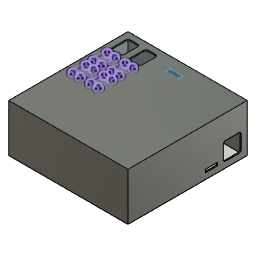
Outer+Hull (Autodesk Fusion 360 design; units mm, degrees)
Autodesk Fusion 360 part; units mm, degrees
sketch "Sketch1" plane through (0, 0, 0) normal (0, 1, 0) x (1, 0, 0) in component "Outer Hull"
  line L0 (0, 0) -> (100, 0)
  line L1 (100, 0) -> (100, -100)
  line L2 (100, -100) -> (0, -100)
  line L3 (0, -100) -> (0, 0)
  dimension "d1" = 100
  dimension "d2" = 100
  constraint horizontal L0
  constraint vertical L1
  constraint horizontal L2
  constraint vertical L3
  constraint coincident L0.start L3.end
  measures "d1" distance of L0.start L0.end
  measures "d2" distance of L0.start L2.end
extrude "Extrude1" add sketch "Sketch1" along normal blind 40 in component "Outer Hull"
shell "Shell1" thickness 1 removed faces 1 at (33.3333, 0, 33.3333) in component "Outer Hull"
sketch "Button hole" plane through (0, 40, 0) normal (0, 1, 0) x (-1, 0, 0)
  line L0 (0, 100) -> (-100, 100)
  line L1 (-100, 100) -> (-100, 0)
  line L2 (-100, 0) -> (0, 0)
  line L3 (0, 0) -> (0, 100)
  line L4 (-7, 5) -> (-13, 5)
  line L5 (-15, 7) -> (-15, 18)
  line L6 (-13, 20) -> (-7, 20)
  line L7 (-5, 18) -> (-5, 7)
  arc A0 (-7, 5) -> (-5, 7) centre (-7, 7) ccw
  arc A1 (-15, 7) -> (-13, 5) centre (-13, 7) ccw
  arc A2 (-13, 20) -> (-15, 18) centre (-13, 18) ccw
  arc A3 (-5, 18) -> (-7, 20) centre (-7, 18) ccw
  dimension "d6" = 2
  constraint horizontal L4
  constraint vertical L5
  constraint horizontal L6
  constraint vertical L7
  constraint tangent L4 A0
  constraint tangent L7 A0
  constraint tangent L4 A1
  constraint tangent L5 A1
  constraint equal A0 A1
  constraint tangent L5 A2
  constraint tangent L6 A2
  constraint equal A0 A2
  constraint tangent L6 A3
  constraint tangent L7 A3
  constraint equal A0 A3
  measures "d6" radius of A0
extrude "Extrude2" cut sketch "Button hole" against normal blind 1 contours L4 L5 L6 L7 A0 A1 A2 A3 in component "Outer Hull"
pattern_linear "R-Pattern1" count 3 spacing 17.5 along (0, 0, 1) count 2 spacing 15 along (1, 0, 0) of "Extrude2" in component "Outer Hull"
sketch "Top toggle" plane through (0, 40, 0) normal (0, 1, 0) x (-1, 0, 0)
  line L0 (-20, 18) -> (-20, 7)
  arc A0 (-22, 5) -> (-20, 7) centre (-22, 7) ccw
  line L1 (-22, 5) -> (-28, 5)
  arc A1 (-30, 7) -> (-28, 5) centre (-28, 7) ccw
  line L2 (-30, 7) -> (-30, 18)
  arc A2 (-28, 20) -> (-30, 18) centre (-28, 18) ccw
  line L3 (-28, 20) -> (-22, 20)
  arc A3 (-20, 18) -> (-22, 20) centre (-22, 18) ccw
  line L4 (-5, 18) -> (-5, 7)
  arc A4 (-7, 5) -> (-5, 7) centre (-7, 7) ccw
  line L5 (-7, 5) -> (-13, 5)
  arc A5 (-15, 7) -> (-13, 5) centre (-13, 7) ccw
  line L6 (-15, 7) -> (-15, 18)
  arc A6 (-13, 20) -> (-15, 18) centre (-13, 18) ccw
  line L7 (-13, 20) -> (-7, 20)
  arc A7 (-5, 18) -> (-7, 20) centre (-7, 18) ccw
  line L8 (0, 100) -> (-100, 100)
  line L9 (-100, 100) -> (-100, 0)
  line L10 (-100, 0) -> (0, 0)
  line L11 (0, 0) -> (0, 100)
  line L12 (-45, 10) -> (-55, 10)
  line L13 (-55, 10) -> (-55, 12.5)
  line L14 (-55, 12.5) -> (-45, 12.5)
  line L15 (-45, 12.5) -> (-45, 10)
  line L16 (-20, 53) -> (-20, 42)
  arc A8 (-22, 40) -> (-20, 42) centre (-22, 42) ccw
  line L17 (-22, 40) -> (-28, 40)
  arc A9 (-30, 42) -> (-28, 40) centre (-28, 42) ccw
  line L18 (-30, 42) -> (-30, 53)
  arc A10 (-28, 55) -> (-30, 53) centre (-28, 53) ccw
  line L19 (-28, 55) -> (-22, 55)
  arc A11 (-20, 53) -> (-22, 55) centre (-22, 53) ccw
  line L20 (-20, 35.5) -> (-20, 24.5)
  arc A12 (-22, 22.5) -> (-20, 24.5) centre (-22, 24.5) ccw
  line L21 (-22, 22.5) -> (-28, 22.5)
  arc A13 (-30, 24.5) -> (-28, 22.5) centre (-28, 24.5) ccw
  line L22 (-30, 24.5) -> (-30, 35.5)
  arc A14 (-28, 37.5) -> (-30, 35.5) centre (-28, 35.5) ccw
  line L23 (-28, 37.5) -> (-22, 37.5)
  arc A15 (-20, 35.5) -> (-22, 37.5) centre (-22, 35.5) ccw
  line L24 (-5, 53) -> (-5, 42)
  arc A16 (-7, 40) -> (-5, 42) centre (-7, 42) ccw
  line L25 (-7, 40) -> (-13, 40)
  arc A17 (-15, 42) -> (-13, 40) centre (-13, 42) ccw
  line L26 (-15, 42) -> (-15, 53)
  arc A18 (-13, 55) -> (-15, 53) centre (-13, 53) ccw
  line L27 (-13, 55) -> (-7, 55)
  arc A19 (-5, 53) -> (-7, 55) centre (-7, 53) ccw
  line L28 (-5, 35.5) -> (-5, 24.5)
  arc A20 (-7, 22.5) -> (-5, 24.5) centre (-7, 24.5) ccw
  line L29 (-7, 22.5) -> (-13, 22.5)
  arc A21 (-15, 24.5) -> (-13, 22.5) centre (-13, 24.5) ccw
  line L30 (-15, 24.5) -> (-15, 35.5)
  arc A22 (-13, 37.5) -> (-15, 35.5) centre (-13, 35.5) ccw
  line L31 (-13, 37.5) -> (-7, 37.5)
  arc A23 (-5, 35.5) -> (-7, 37.5) centre (-7, 35.5) ccw
  dimension "d17" = 10
  dimension "d18" = 2.5
  constraint horizontal L12
  constraint vertical L13
  constraint horizontal L14
  constraint vertical L15
  measures "d17" distance of L12.start L12.end
  measures "d18" distance of L12.start L14.end
extrude "Extrude3" cut sketch "Top toggle" against normal blind 1 contours L12 L13 L14 L15 in component "Outer Hull"
sketch "Wire inlet" plane through (100, 0, 0) normal (1, 0, 0) x (0, 0, -1)
  line L0 (-100, 0) -> (0, 0)
  line L1 (0, 0) -> (0, 40)
  line L2 (0, 40) -> (-100, 40)
  line L3 (-100, 40) -> (-100, 0)
  line L4 (-7, 5) -> (-18, 5)
  line L5 (-20, 7) -> (-20, 18)
  line L6 (-18, 20) -> (-7, 20)
  line L7 (-5, 18) -> (-5, 7)
  arc A0 (-18, 20) -> (-20, 18) centre (-18, 18) ccw
  arc A1 (-5, 18) -> (-7, 20) centre (-7, 18) ccw
  arc A2 (-7, 5) -> (-5, 7) centre (-7, 7) ccw
  arc A3 (-20, 7) -> (-18, 5) centre (-18, 7) ccw
  dimension "d21" = 2
  constraint horizontal L4
  constraint vertical L5
  constraint horizontal L6
  constraint vertical L7
  constraint tangent L5 A0
  constraint tangent L6 A0
  constraint tangent L6 A1
  constraint tangent L7 A1
  constraint equal A0 A1
  constraint tangent L4 A2
  constraint tangent L7 A2
  constraint equal A0 A2
  constraint tangent L4 A3
  constraint tangent L5 A3
  constraint equal A0 A3
  measures "d21" radius of A0
extrude "Extrude4" cut sketch "Wire inlet" against normal blind 1 contours L4 L5 L6 L7 A0 A1 A2 A3 in component "Outer Hull"
sketch "Sketch4" plane through (100, 0, 0) normal (1, 0, 0) x (0, 0, -1)
  line L0 (-20, 7) -> (-20, 18)
  arc A0 (-18, 20) -> (-20, 18) centre (-18, 18) ccw
  line L1 (-18, 20) -> (-7, 20)
  arc A1 (-5, 18) -> (-7, 20) centre (-7, 18) ccw
  line L2 (-5, 18) -> (-5, 7)
  arc A2 (-7, 5) -> (-5, 7) centre (-7, 7) ccw
  line L3 (-7, 5) -> (-18, 5)
  arc A3 (-20, 7) -> (-18, 5) centre (-18, 7) ccw
  line L4 (-100, 0) -> (0, 0)
  line L5 (0, 0) -> (0, 40)
  line L6 (0, 40) -> (-100, 40)
  line L7 (-100, 40) -> (-100, 0)
  line L8 (-25, 5) -> (-35, 5)
  line L9 (-35, 5) -> (-35, 7.5)
  line L10 (-35, 7.5) -> (-25, 7.5)
  line L11 (-25, 7.5) -> (-25, 5)
  dimension "d24" = 10
  dimension "d25" = 2.5
  constraint horizontal L8
  constraint vertical L9
  constraint horizontal L10
  constraint vertical L11
  measures "d24" distance of L8.start L8.end
  measures "d25" distance of L8.start L10.end
extrude "Extrude5" cut sketch "Sketch4" against normal blind 1 contours L8 L9 L10 L11 in component "Outer Hull"
component "Outer Hull" placed x (1, 0, 0) y (0, 1, 0) z (0, 0, 1) at (0, 0, 0)
